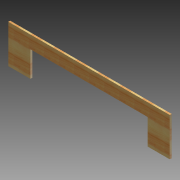
# Autodesk Inventor part: plywood front pannel 2
Saved by Autodesk Inventor 2012 (Build 160160000, 160)
## iProperties
Created: 2013-10-07
Part Number: plywood front pannel 2
Material: Default
Document SubType Name: Modeling
Designer: Bryce
Density: 1 g/cm^3
Author: Bryce
Autodesk Inventor part; units mm, degrees
ref_plane "YZ Plane" through (0, 0, 0) normal (1, 0, 0) x (0, 1, 0)
ref_plane "XZ Plane" through (0, 0, 0) normal (0, 1, 0) x (-1, 0, 0)
ref_plane "XY Plane" through (0, 0, 0) normal (0, 0, 1) x (1, 0, 0)
sketch "Sketch1" plane through (0, 0, 0) normal (0, 0, 1) x (1, 0, 0)
  line L0 (962.025, 0) -> (962.025, 228.6)
  line L1 (962.025, 228.6) -> (0, 228.6)
  line L2 (0, 228.6) -> (0, 0)
  line L3 (830.2625, 0) -> (830.2625, 152.4)
  line L4 (830.2625, 152.4) -> (131.7625, 152.4)
  line L5 (131.7625, 152.4) -> (131.7625, 0)
  line L6 (0, 0) -> (131.7625, 0)
  line L7 (830.2625, 0) -> (962.025, 0)
  dimension "d0" = 962.025
  dimension "d1" = 228.6
  dimension "d2" = 698.5
  dimension "d3" = 131.7625
  dimension "d4" = 131.7625
  dimension "d5" = 76.2
  constraints: 16 end point, 4 parallel, 2 horizontal, 2 perpendicular, 1 collinear
  measures "d0" distance of L2.end L0.start
  measures "d1" distance of L1.end L2.end
  measures "d2" distance of L3.end L4.end
  measures "d3" distance between parallel lines of L2 L5
  measures "d4" distance between parallel lines of L0 L3
  measures "d5" distance between parallel lines of L1 L4
extrude "Extrusion1" add sketch "Sketch1" along normal blind 11.1125
equation "\"d3\" = d4"
body "Solid1"
